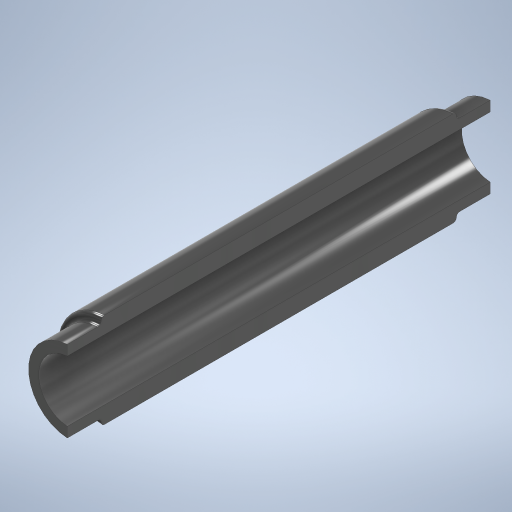
# Autodesk Inventor part: handle
Saved by Autodesk Inventor 2023.4 (Build 274418000, 418)
## iProperties
Created: 2024-01-29
Part Number: handle
Material: Generic
Document SubType Name: Modeling
Designer: aaron
Density: 1 g/cm^3
Appearance: Default
Author: aaron
Autodesk Inventor part; units mm, degrees
ref_plane "YZ Plane" through (0, 0, 0) normal (1, 0, 0) x (0, 1, 0)
ref_plane "XZ Plane" through (0, 0, 0) normal (0, 1, 0) x (-1, 0, 0)
ref_plane "XY Plane" through (0, 0, 0) normal (0, 0, 1) x (1, 0, 0)
sketch "Sketch1" plane through (0, 0, 0) normal (0, 0, 1) x (1, 0, 0)
  circle A0 centre (0, 0) radius 14
  dimension "d0" = 28
  constraints: 1 centre point, 1 coincident
  measures "d0" diameter of A0
extrude "Extrusion1" add sketch "Sketch1" against normal blind 105
sketch "Sketch2" plane through (0, 0, 0) normal (0, 0, 1) x (1, 0, 0)
  circle A0 centre (0, 0) radius 14 projected
  circle A1 centre (0, 0) radius 12
  dimension "d3" = 2
  constraints: 1 centre point
  measures "d3" radial gap between concentric circles of A0 A1
extrude "Extrusion2" add sketch "Sketch2" along normal blind 10 contours A1
sketch "Sketch3" plane through (0, 0, -105) normal (0, 0, -1) x (-1, 0, 0)
  circle A0 centre (0, 0) radius 12 projected
extrude "Extrusion3" add sketch "Sketch3" along normal blind 10
fillet "Fillet1" radius 1 4 edges at (-12, 0, 0) (-14, 0, 0) (-14, 0, -105) (12, 0, -105)
sketch "Sketch4" plane through (0, 0, 10) normal (0, 0, 1) x (1, 0, 0)
  circle A0 centre (0, 0) radius 12 projected
  circle A1 centre (0, 0) radius 9
  dimension "d9" = 3
  constraints: 1 centre point
  measures "d9" radial gap between concentric circles of A0 A1
extrude "Extrusion4" cut sketch "Sketch4" against normal through all contours A1
sketch "Sketch5" plane through (0, 0, 10) normal (0, 0, 1) x (1, 0, 0)
  line L0 (0, -18.4925) -> (0, 18.8644)
  line L1 (-0.55, -18.4925) -> (-0.55, 18.8644)
  line L2 (-0.55, -18.4925) -> (-0.55, -24.6298)
  line L3 (-0.55, -24.6298) -> (18.7736, -14.0631)
  line L4 (18.7736, -14.0631) -> (17.813, 9.6853)
  line L5 (17.813, 9.6853) -> (0, 24.9482)
  line L6 (0, 24.9482) -> (-0.55, 18.8644)
  point P0 (0, 0)
  dimension "d12" = 0.55
  constraints: 14 end point, 2 vertical, 1 parallel
  measures "d12" distance between parallel lines of L0 L1
extrude "Extrusion5" cut sketch "Sketch5" against normal through all
body "Solid1"
